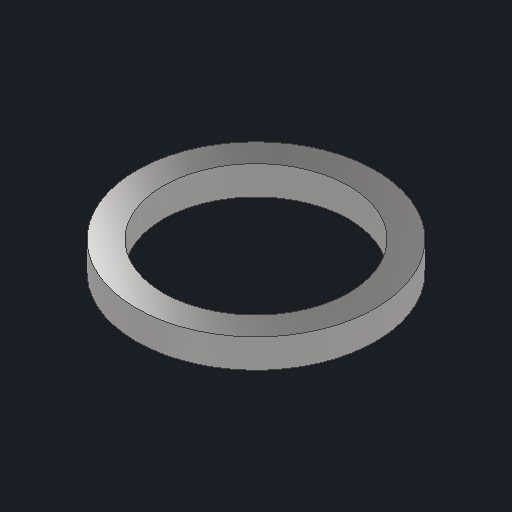
# Autodesk Inventor part: Case_Bearing_GB
Saved by Autodesk Inventor 2024.2 (Build 282272000, 272)
## iProperties
Created: 2026-01-04
Part Number: Case_Bearing_GB
Material: Stainless Steel
Document SubType Name: Modeling
Designer: 4aida
Density: 8 g/cm^3
Appearance: Semi-Polished
Author: 4aida
Autodesk Inventor part; units mm, degrees
ref_plane "YZ Plane" through (0, 0, 0) normal (1, 0, 0) x (0, 1, 0)
ref_plane "XZ Plane" through (0, 0, 0) normal (0, 1, 0) x (-1, 0, 0)
ref_plane "XY Plane" through (0, 0, 0) normal (0, 0, 1) x (1, 0, 0)
sketch "Sketch1" plane through (0, 0, 0) normal (1, 0, 0) x (0, 1, 0)
  line L0 (-3.5, 22.5) -> (3.5, 22.5)
  line L1 (3.5, 22.5) -> (3.5, 29)
  line L2 (3.5, 29) -> (-3.5, 29)
  line L3 (-3.5, 29) -> (-3.5, 22.5)
  line L4 (-3.5, 22.5) -> (3.5, 29) construction
  line L5 (3.5, 22.5) -> (-3.5, 29) construction
  line L6 (3.5, 0) -> (-3.5, 0)
  point P0 (0, 0)
  point P1 (0, 25.75)
  point P2 (0, 0)
  dimension "d0" = 45
  dimension "d1" = 58
  dimension "d2" = 7
  constraints: 14 end point, 3 midpoint, 2 horizontal, 2 parallel, 2 vertical alignment, 1 coincident, 1 perpendicular
  measures "d0" diameter of L0 L6
  measures "d1" diameter of L2 L6
  measures "d2" distance of L1.end L2.end
revolve "Revolution1" add sketch "Sketch1" angle 360 about axis through (0, 3.5, 0) along (0, -1, 0)
body "Solid1"
